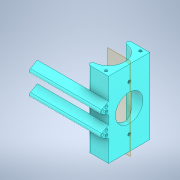
# Autodesk Inventor part: Tubo Exterior
Saved by Autodesk Inventor 2020.3 (Build 243373000, 373)
## iProperties
Created: 2020-07-26
Part Number: Tubo Exterior
Material: ABS Plastic
Document SubType Name: Modeling
Designer: juanp
Density: 1.06 g/cm^3
Appearance: Smooth - White
Author: juanp
Autodesk Inventor part; units mm, degrees
ref_plane "YZ Plane" through (0, 0, 0) normal (1, 0, 0) x (0, 1, 0)
ref_plane "XZ Plane" through (0, 0, 0) normal (0, 1, 0) x (-1, 0, 0)
ref_plane "XY Plane" through (0, 0, 0) normal (0, 0, 1) x (1, 0, 0)
sketch "Sketch1" plane through (0, 0, 0) normal (0, 1, 0) x (-1, 0, 0)
  arc A0 (0, 30.16) -> (-3.6283, 29.941) centre (0, 0) ccw construction
  arc A1 (-26.9832, 26.9832) -> (-36.0277, -12.5774) centre (0, 0) ccw construction
  line L0 (38.16, 38.16) -> (0, 38.16) construction
  line L1 (-38.16, 38.16) -> (-38.16, -38.16)
  line L2 (-38.16, -38.16) -> (-4.1245, -38.16)
  line L3 (38.16, -38.16) -> (38.16, 38.16) construction
  line L4 (38.16, 38.16) -> (-21.3263, -21.3263) construction
  line L5 (-38.16, 38.16) -> (-21.3263, 21.3263) construction
  line L6 (0, 38.16) -> (-4.1245, 38.16) construction
  line L7 (0, -38.16) -> (38.16, -38.16) construction
  arc A2 (0, 38.16) -> (-26.9832, 26.9832) centre (0, 0) ccw construction
  arc A3 (-36.9415, -9.566) -> (-26.9832, -26.9832) centre (0, 0) ccw construction
  arc A4 (-26.9832, -26.9832) -> (0, -38.16) centre (0, 0) ccw construction
  arc A5 (0, -38.16) -> (0, 38.16) centre (0, 0) ccw construction
  line L8 (-21.3263, 21.3263) -> (38.16, -38.16) construction
  line L9 (-21.3263, -21.3263) -> (-38.16, -38.16) construction
  line L10 (0, 38.16) -> (0, 30.16) construction
  line L11 (0, -30.16) -> (0, -38.16) construction
  arc A6 (21.3263, 21.3263) -> (0, 30.16) centre (0, 0) ccw construction
  arc A7 (0, -30.16) -> (21.3263, 21.3263) centre (0, 0) ccw construction
  arc A8 (-6.0651, -37.6749) -> (-3.6283, -29.941) centre (-4.1245, -34.0355) ccw
  arc A9 (-3.6283, 29.941) -> (-6.0651, 37.6749) centre (-4.1245, 34.0355) ccw
  line L12 (-4.1245, -38.16) -> (0, -38.16) construction
  arc A10 (-3.6283, -29.941) -> (0, -30.16) centre (0, 0) ccw construction
  arc A11 (-3.6283, 29.941) -> (-3.6283, -29.941) centre (0, 0) ccw
  line L13 (-4.1245, 38.16) -> (-38.16, 38.16)
  arc A12 (-3.6283, -29.941) -> (-6.0651, -37.6749) centre (-4.1245, -34.0355) ccw construction
  arc A13 (-6.0651, 37.6749) -> (-3.6283, 29.941) centre (-4.1245, 34.0355) ccw construction
  dimension "d0" = 60.32
  dimension "d1" = 8
  constraints: 42 point on circle, 28 end point, 21 tangent, 14 centre point, 10 parallel, 8 point on line, 3 horizontal, 3 perpendicular, 2 coincident, 1 vertical
  measures "d0" diameter of A0
  measures "d1" radial gap between concentric circles of A1 A0
extrude "Extrusion1" add sketch "Sketch1" along normal blind 140
sketch "Sketch2" plane through (38.16, 0, 38.16) normal (1, 0, 0) x (0, 0, -1)
  line L0 (8.219, 140) -> (0, 140) projected
  line L1 (0, 140) -> (76.32, 0) construction
  line L2 (76.32, 140) -> (0, 0) construction
  circle A0 centre (38.16, 70) radius 25.4
  dimension "d15" = 50.8
  constraints: 4 end point, 1 centre point, 1 midpoint
  measures "d15" diameter of A0
extrude "Extrusion2" cut sketch "Sketch2" against normal up to next
ref_plane "Work Plane1" through (0, 70, 0) normal (0, 1, 0) x (1, 0, 0)
sketch "Sketch3" plane through (0, 70, 0) normal (0, 1, 0) x (1, 0, 0)
  line L0 (38.16, 38.16) -> (4.1245, 38.16) projected
  line L1 (38.16, 25.4) -> (16.2624, 25.4) projected
  line L2 (38.16, -38.16) -> (38.16, 38.16) projected
  line L3 (38.16, -25.4) -> (16.2624, -25.4) projected
  line L4 (4.1245, -38.16) -> (38.16, -38.16) projected
  line L5 (16.2624, 25.4) -> (38.16, 38.16) construction
  line L6 (38.16, 25.4) -> (16.2624, 38.16) construction
  line L7 (16.2624, -25.4) -> (38.16, -38.16) construction
  line L8 (38.16, -25.4) -> (16.2624, -38.16) construction
  circle A0 centre (27.2112, 31.78) radius 2.5
  circle A1 centre (27.2112, -31.78) radius 2.5
  dimension "d16" = 5
  dimension "d17" = 5
  constraints: 8 end point, 2 centre point, 2 midpoint, 2 parallel, 2 point on line
  measures "d16" diameter of A0
  measures "d17" diameter of A1
extrude "Extrusion3" cut sketch "Sketch3" along normal through all both and the other way through all
sketch "Sketch5" plane through (38.16, 0, 38.16) normal (1, 0, 0) x (0, 0, -1)
  circle A0 centre (38.16, 70) radius 25.4 projected
  line L0 (0, 140) -> (76.32, 140) projected
  line L1 (0, 0) -> (76.32, 0) projected
  line L2 (38.16, 95.4) -> (38.16, 140) construction
  line L3 (38.16, 44.6) -> (38.16, 0) construction
  circle A1 centre (38.16, 112.125) radius 2.55
  circle A2 centre (38.16, 27.875) radius 2.55
  line L4 (38.16, 22.3) -> (38.16, 44.6) construction
  line L5 (38.16, 117.7) -> (38.16, 95.4) construction
  line L6 (38.16, 22.3) -> (38.16, 33.45)
  line L7 (38.16, 117.7) -> (38.16, 106.55)
  dimension "d18" = 5.1
  dimension "d19" = 5.1
  constraints: 12 end point, 7 midpoint, 3 collinear, 2 centre point, 2 coincident, 2 point on circle, 1 point on line
  measures "d18" diameter of A1
  measures "d19" diameter of A2
extrude "Extrusion4" cut sketch "Sketch5" against normal up to next contours A1 L7 | L7 A1 | A2 L6 | L6 A2
ref_plane "Work Plane2" through (4.1245, 0, 0) normal (0, 0, 1) x (1, 0, 0)
sketch "Sketch7" plane through (38.16, 0, 38.16) normal (1, 0, 0) x (0, 0, -1)
  line L0 (0, 0) -> (0, 140) construction
  line L1 (0, 140) -> (0, 0) construction
  line L2 (0, 89) -> (0, 51)
  circle A0 centre (-4, 93) radius 4 construction
  circle A1 centre (-4, 93) radius 2.75
  circle A2 centre (-4, 85) radius 4 construction
  circle A3 centre (-4, 85) radius 2.75
  arc A4 (-12.9282, 85.5359) -> (-12.9282, 92.4641) centre (-10.9282, 89) ccw construction
  circle A5 centre (-10.9282, 89) radius 2.75
  line L3 (0, 70) -> (-10, 70) construction
  line L4 (0, 89) -> (-10, 89) construction
  line L5 (0, 78.0718) -> (-12.9282, 85.5359)
  line L6 (-12.9282, 92.4641) -> (0, 99.9282)
  arc A6 (-12.9282, 92.4641) -> (-12.9282, 85.5359) centre (-10.9282, 89) ccw
  circle A7 centre (-4, 47) radius 4 construction
  circle A8 centre (-4, 47) radius 2.75
  circle A9 centre (-4, 55) radius 4 construction
  circle A10 centre (-4, 55) radius 2.75
  arc A11 (-12.9282, 47.5359) -> (-12.9282, 54.4641) centre (-10.9282, 51) ccw construction
  circle A12 centre (-10.9282, 51) radius 2.75
  line L7 (0, 51) -> (-10, 51) construction
  line L8 (0, 61.9282) -> (-12.9282, 54.4641)
  line L9 (-12.9282, 47.5359) -> (0, 40.0718)
  arc A13 (-12.9282, 54.4641) -> (-12.9282, 47.5359) centre (-10.9282, 51) ccw
  line L10 (0, 89) -> (0, 99.9282)
  line L11 (0, 51) -> (0, 40.0718)
  point P0 (38.16, 0)
  dimension "d26" = 38
  dimension "d27" = 8
  dimension "d28" = 5.5
  dimension "d29" = 8
  dimension "d30" = 5.5
  dimension "d31" = 8
  dimension "d32" = 5.5
  dimension "d33" = 10
  dimension "d34" = 10
  constraints: 22 end point, 14 centre point, 11 symmetric about line, 10 tangent, 8 point on circle, 6 coincident, 2 collinear, 2 midpoint, 2 point on line, 2 vertical, 1 horizontal, 1 perpendicular, 7 other
  measures "d26" distance of L2.start L2.end
  measures "d27" diameter of A0
  measures "d28" diameter of A1
  measures "d29" diameter of A2
  measures "d30" diameter of A3
  measures "d31" diameter of A4
  measures "d32" diameter of A5
  measures "d33" distance of L3.start L3.end
  measures "d34" distance of L2.start L4.end
extrude "Extrusion6" add sketch "Sketch7" against normal blind 132
body "Solid1"
